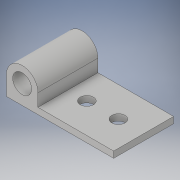
# Autodesk Inventor part: PKWS1_b
Saved by Autodesk Inventor 2019 (Build 230136000, 136)
## iProperties
Created: 2024-01-04
Part Number: PKWS1_b
Material: Generic
Catalog Web Link: www.cadenas.de
Description: PKWS_base-Snap Locks
Vendor: MISUMI
Document SubType Name: Modeling
Designer: psAdmin
Manufacturer: MISUMI
Mass: 0.275687 g
Surface Area: 5.55486 cm^2
Volume: 0.275687 cm^3
Density: 1 g/cm^3
Appearance: PSOLRGB-175-175-175
Category: PARTsolutions
Company: MISUMI
Title: PKWS1
Author: Cadenas PARTsolutions
Comments: Snap Locks
PSOL_IDENT_0: {$CADENAS_DATA/23d-libs/misumi/metric/44_handles_hinges/pkws_base.prj},155 {VTYP=3D},{NB=PKWS1_b},{L
PSOL_IDENT_1: INA=PKWS1},{NN=PKWS_base},{DATE=17.04.2023 00:27:41},{GEOMDATE=04.04.2023 01:08:01},{VERSION=},{LINE
PSOL_IDENT_2: ID=10},{WBVAR=},{WBNUMERIC=}  {NB=PKWS1_b},{LINA=PKWS1},{KT=DUMMY},{PN=PKWS1},{NO=1},{TL=49 (5)},{MA
PSOL_IDENT_3: SS=11},{PPATH=assemblies_pkws\\pkws_templ.prj},{ANGLE=10.015}
NB: PKWS1_b
NN: PKWS_base
NT: Snap Locks
NBSYN: $PN._b
LINA: PKWS1
CATALOG: Misumi
PN: PKWS1
NO: 1
TL: 49 (5)
MASS: 11
SUPPLIER: MISUMI
ARTICLENO: PKWS1_b
BOMINFO: PKWS1
CREATOR: CADENAS GmbH
Autodesk Inventor part; units mm, degrees
sketch "Sketch_1" plane through (0, 0, 0) normal (0, 0, 1) x (1, 0, 0)
  line L0 (0, 3) -> (0, 0)
  line L1 (0, 0) -> (17, 0)
  line L2 (17, 0) -> (17, 1)
  line L3 (17, 1) -> (5, 1)
  line L4 (5, 1) -> (5, 3)
  arc A0 (5, 3) -> (0, 3) centre (2.5, 3) ccw
  circle A1 centre (2.5, 3) radius 1.5
  constraints: 10 end point, 2 centre point, 2 point on circle
extrude "Extrusion1" add sketch "Sketch_1" along normal mid plane 9.5
sketch "Sketch_2" plane through (0, 0, 0) normal (0, 1, 0) x (-1, 0, 0)
  circle A0 centre (-8, 0) radius 1.05
  constraints: 1 centre point
extrude "Extrusion2" cut sketch "Sketch_2" along normal mid plane 9.5
sketch "Sketch_3" plane through (0, 0, 0) normal (0, 1, 0) x (-1, 0, 0)
  circle A0 centre (-13, 0) radius 1.05
  constraints: 1 centre point
extrude "Extrusion3" cut sketch "Sketch_3" along normal mid plane 9.5
ref_plane "A_XY" through (2.5, 3, 0) normal (0, 0, 1) x (1, 0, 0)
ref_plane "A_YZ" through (2.5, 3, 0) normal (1, 0, 0) x (0, 1, 0)
ref_plane "A_ZX" through (2.5, 3, 0) normal (0, 1, 0) x (0, 0, 1)
body "Solid1"
